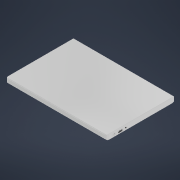
# Autodesk Inventor part: Razor Book 13
Saved by Autodesk Inventor 2021.3 (Build 253353000, 353)
## iProperties
Created: 2021-04-25
Part Number: Razor Book 13
Material: Generic
Document SubType Name: Modeling
Designer: trl121
Density: 1 g/cm^3
Appearance: Default
Author: trl121
Autodesk Inventor part; units mm, degrees
ref_plane "YZ Plane" through (0, 0, 0) normal (1, 0, 0) x (0, 1, 0)
ref_plane "XZ Plane" through (0, 0, 0) normal (0, 1, 0) x (-1, 0, 0)
ref_plane "XY Plane" through (0, 0, 0) normal (0, 0, 1) x (1, 0, 0)
sketch "Base" plane through (0, 0, 0) normal (0, 1, 0) x (-1, 0, 0)
  line L0 (-147.8, 99.5763) -> (147.8, 99.5763) construction
  line L1 (147.8, 99.5763) -> (147.8, -99.5763) construction
  line L2 (147.8, -99.5763) -> (-147.8, -99.5763) construction
  line L3 (-147.8, -99.5763) -> (-147.8, 99.5763) construction
  line L4 (-147.8, 99.5763) -> (147.8, 99.5763)
  line L5 (147.8, 99.5763) -> (147.8, -99.5763)
  line L6 (147.8, -99.5763) -> (-147.8, -99.5763)
  line L7 (-147.8, -99.5763) -> (-147.8, 99.5763)
  line L8 (-147.8, 99.5763) -> (147.8, -99.5763) construction
  line L9 (147.8, 99.5763) -> (-147.8, -99.5763) construction
  point P0 (0, 0)
  point P1 (0, 0)
  point P2 (0, 0)
  dimension "d2" = 295.6
  dimension "d6" = 199.1527
  constraints: 12 end point, 3 midpoint, 2 coincident, 2 horizontal, 2 parallel, 1 perpendicular, 2 other
  measures "d2" distance between parallel lines of L3 L1
  measures "d6" distance of L2.end L0.start
sketch "Side" plane through (0, 0, 0) normal (1, 0, 0) x (0, 1, 0)
  line L0 (0, -99.5763) -> (0, 99.5763) construction
  line L1 (7.8769, 99.5763) -> (7.8769, -99.5763) construction
  line L2 (7.8769, -99.5763) -> (-7.8769, -99.5763) construction
  line L3 (-7.8769, -99.5763) -> (-7.8769, 99.5763) construction
  line L4 (-7.8769, 99.5763) -> (7.8769, 99.5763) construction
  line L5 (7.8769, 99.5763) -> (-7.8769, 99.5763) construction
  line L6 (-7.8769, 99.5763) -> (-7.8769, -99.5763) construction
  line L7 (-7.8769, -99.5763) -> (7.8769, -99.5763) construction
  line L8 (7.8769, -99.5763) -> (7.8769, 99.5763) construction
  line L9 (6.5964, 99.5763) -> (6.5964, 98.1719)
  line L10 (6.5964, 98.1719) -> (7.8769, 98.1719)
  line L11 (-3.3255, 99.5763) -> (-3.3255, 98.1719)
  line L12 (-3.3255, 98.1719) -> (-4.3415, 98.1719)
  ellipse E0 centre (-4.3415, 88.4565) end of major axis (-4.3415, 98.1719) minor radius 2.4965 (-4.3415, 98.1719) -> (-6.838, 88.4565) ccw
  line L13 (-6.838, 88.4565) -> (-6.838, 75.8385)
  line L14 (6.5964, 99.5763) -> (-3.3255, 99.5763)
  ellipse E1 centre (-6.838, 74.0859) end of major axis (-6.838, 75.8385) minor radius 1.0389 (-6.838, 75.8385) -> (-7.8769, 74.0859) ccw
  line L15 (-6.838, 75.8385) -> (-6.308, 75.8385) construction
  line L16 (-7.8769, 74.0859) -> (-7.8769, 69.5647)
  line L17 (-7.8769, 71.8253) -> (-6.4493, 71.8253) construction
  ellipse E2 centre (-6.838, 69.5647) end of major axis (-6.838, 67.8121) minor radius 1.0389 (-7.8769, 69.5647) -> (-6.838, 67.8121) ccw
  line L18 (-6.838, 75.8385) -> (-6.838, 67.8121)
  line L19 (-6.838, 67.8121) -> (-6.838, -69.2956)
  line L20 (-6.838, -0.7418) -> (-5.3966, -0.7418) construction
  ellipse E3 centre (-6.838, -75.5694) end of major axis (-6.838, -77.322) minor radius 1.0389 (-7.8769, -75.5694) -> (-6.838, -77.322) ccw
  line L21 (-7.8769, -75.5694) -> (-7.8769, -71.0482)
  ellipse E4 centre (-6.838, -71.0482) end of major axis (-6.838, -69.2956) minor radius 1.0389 (-6.838, -69.2956) -> (-7.8769, -71.0482) ccw
  line L22 (-6.838, -77.322) -> (-6.838, -69.2956)
  line L23 (7.8769, 98.1719) -> (7.8769, -99.0683)
  line L24 (7.3689, -99.5763) -> (-4.2591, -99.5763)
  line L25 (-6.838, -77.322) -> (-6.838, -91.1477)
  ellipse E5 centre (-4.2591, -91.1477) end of major axis (-4.2591, -99.5763) minor radius 2.5789 (-6.838, -91.1477) -> (-4.2591, -99.5763) ccw
  arc A0 (7.3689, -99.5763) -> (7.8769, -99.0683) centre (7.3689, -99.0683) ccw
  point P0 (0, 0)
  point P1 (-5.6451, -98.2557)
  dimension "d42" = 1.016
  dimension "d82" = 1.7526
  dimension "d90" = 8.0264
  dimension "d119" = 0.508
  constraints: 42 end point, 13 horizontal, 11 point on line, 7 symmetric about line, 7 vertical, 6 perpendicular, 4 midpoint, 3 parallel, 2 collinear, 2 point on circle, 2 tangent, 1 centre point, 1 horizontal alignment, 28 other
  measures "d42" distance of L11.end L12.end
  measures "d82" distance from line of L15 point (-6.838, 74.086)
  measures "d90" distance from line of L18.end L15
  measures "d119" radius of A0
extrude "Main Body" add sketch "Side" along normal mid plane 295.6 contours L9 L10 L23 A0 L24 E5 L25 L22 L19 L18 L13 E0 L12 L11 L14
sketch "Bottom" plane through (-147.8, -6.838, -91.1477) normal (0, -1, 0) x (1, 0, 0)
  line L0 (0, 190.724) -> (295.6, 190.724) construction
  line L1 (295.6, 190.724) -> (295.6, 44.5306) construction
  line L2 (295.6, 44.5306) -> (0, 44.5306) construction
  line L3 (0, 44.5306) -> (0, 190.724) construction
  line L4 (295.6, 179.6042) -> (295.6, 0) projected
  line L5 (27.94, 140.178) -> (72.39, 140.178)
  line L6 (73.66, 138.908) -> (73.66, 135.606)
  line L7 (72.39, 134.336) -> (27.94, 134.336)
  line L8 (26.67, 135.606) -> (26.67, 138.908)
  arc A0 (27.94, 140.178) -> (26.67, 138.908) centre (27.94, 138.908) ccw
  arc A1 (26.67, 135.606) -> (27.94, 134.336) centre (27.94, 135.606) ccw
  arc A2 (73.66, 138.908) -> (72.39, 140.178) centre (72.39, 138.908) ccw
  arc A3 (72.39, 134.336) -> (73.66, 135.606) centre (72.39, 135.606) ccw
  line L9 (27.94, 130.78) -> (72.39, 130.78)
  arc A4 (27.94, 130.78) -> (26.67, 129.51) centre (27.94, 129.51) ccw
  line L10 (26.67, 126.208) -> (26.67, 129.51)
  arc A5 (26.67, 126.208) -> (27.94, 124.938) centre (27.94, 126.208) ccw
  line L11 (72.39, 124.938) -> (27.94, 124.938)
  arc A6 (72.39, 124.938) -> (73.66, 126.208) centre (72.39, 126.208) ccw
  line L12 (73.66, 129.51) -> (73.66, 126.208)
  arc A7 (73.66, 129.51) -> (72.39, 130.78) centre (72.39, 129.51) ccw
  line L13 (27.94, 121.382) -> (72.39, 121.382)
  arc A8 (27.94, 121.382) -> (26.67, 120.112) centre (27.94, 120.112) ccw
  line L14 (26.67, 116.81) -> (26.67, 120.112)
  arc A9 (26.67, 116.81) -> (27.94, 115.54) centre (27.94, 116.81) ccw
  line L15 (72.39, 115.54) -> (27.94, 115.54)
  arc A10 (72.39, 115.54) -> (73.66, 116.81) centre (72.39, 116.81) ccw
  line L16 (73.66, 120.112) -> (73.66, 116.81)
  arc A11 (73.66, 120.112) -> (72.39, 121.382) centre (72.39, 120.112) ccw
  line L17 (27.94, 111.984) -> (72.39, 111.984)
  arc A12 (27.94, 111.984) -> (26.67, 110.714) centre (27.94, 110.714) ccw
  line L18 (26.67, 107.412) -> (26.67, 110.714)
  arc A13 (26.67, 107.412) -> (27.94, 106.142) centre (27.94, 107.412) ccw
  line L19 (72.39, 106.142) -> (27.94, 106.142)
  arc A14 (72.39, 106.142) -> (73.66, 107.412) centre (72.39, 107.412) ccw
  line L20 (73.66, 110.714) -> (73.66, 107.412)
  arc A15 (73.66, 110.714) -> (72.39, 111.984) centre (72.39, 110.714) ccw
  line L21 (147.8, 190.724) -> (147.8, 44.5306) construction
  line L22 (267.66, 140.178) -> (223.21, 140.178)
  line L23 (221.94, 138.908) -> (221.94, 135.606)
  line L24 (223.21, 134.336) -> (267.66, 134.336)
  line L25 (268.93, 135.606) -> (268.93, 138.908)
  arc A16 (268.93, 138.908) -> (267.66, 140.178) centre (267.66, 138.908) ccw
  arc A17 (267.66, 134.336) -> (268.93, 135.606) centre (267.66, 135.606) ccw
  arc A18 (223.21, 140.178) -> (221.94, 138.908) centre (223.21, 138.908) ccw
  arc A19 (221.94, 135.606) -> (223.21, 134.336) centre (223.21, 135.606) ccw
  line L26 (267.66, 130.78) -> (223.21, 130.78)
  arc A20 (268.93, 129.51) -> (267.66, 130.78) centre (267.66, 129.51) ccw
  line L27 (268.93, 126.208) -> (268.93, 129.51)
  arc A21 (267.66, 124.938) -> (268.93, 126.208) centre (267.66, 126.208) ccw
  line L28 (223.21, 124.938) -> (267.66, 124.938)
  arc A22 (221.94, 126.208) -> (223.21, 124.938) centre (223.21, 126.208) ccw
  line L29 (221.94, 129.51) -> (221.94, 126.208)
  arc A23 (223.21, 130.78) -> (221.94, 129.51) centre (223.21, 129.51) ccw
  line L30 (267.66, 121.382) -> (223.21, 121.382)
  arc A24 (268.93, 120.112) -> (267.66, 121.382) centre (267.66, 120.112) ccw
  line L31 (268.93, 116.81) -> (268.93, 120.112)
  arc A25 (267.66, 115.54) -> (268.93, 116.81) centre (267.66, 116.81) ccw
  line L32 (223.21, 115.54) -> (267.66, 115.54)
  arc A26 (221.94, 116.81) -> (223.21, 115.54) centre (223.21, 116.81) ccw
  line L33 (221.94, 120.112) -> (221.94, 116.81)
  arc A27 (223.21, 121.382) -> (221.94, 120.112) centre (223.21, 120.112) ccw
  line L34 (267.66, 111.984) -> (223.21, 111.984)
  arc A28 (268.93, 110.714) -> (267.66, 111.984) centre (267.66, 110.714) ccw
  line L35 (268.93, 107.412) -> (268.93, 110.714)
  arc A29 (267.66, 106.142) -> (268.93, 107.412) centre (267.66, 107.412) ccw
  line L36 (223.21, 106.142) -> (267.66, 106.142)
  arc A30 (221.94, 107.412) -> (223.21, 106.142) centre (223.21, 107.412) ccw
  line L37 (221.94, 110.714) -> (221.94, 107.412)
  arc A31 (223.21, 111.984) -> (221.94, 110.714) centre (223.21, 110.714) ccw
  line L38 (0, 190.724) -> (295.6, 190.724) projected
  line L39 (5.08, 190.724) -> (0, 190.724)
  line L40 (0, 190.724) -> (0, 185.644)
  line L41 (0, 189.3196) -> (0, 179.6042) projected
  arc A32 (5.08, 190.724) -> (0, 185.644) centre (5.08, 185.644) ccw
  line L42 (295.6, 190.724) -> (295.6, 185.644)
  arc A33 (295.6, 185.644) -> (290.52, 190.724) centre (290.52, 185.644) ccw
  line L43 (290.52, 190.724) -> (295.6, 190.724)
  line L44 (27.5437, 176.5) -> (32.6237, 176.5)
  line L45 (33.1317, 175.992) -> (33.1317, 172.69)
  line L46 (32.6237, 172.182) -> (27.5437, 172.182)
  line L47 (27.0357, 172.69) -> (27.0357, 175.992)
  arc A34 (27.5437, 176.5) -> (27.0357, 175.992) centre (27.5437, 175.992) ccw
  arc A35 (27.0357, 172.69) -> (27.5437, 172.182) centre (27.5437, 172.69) ccw
  arc A36 (32.6237, 172.182) -> (33.1317, 172.69) centre (32.6237, 172.69) ccw
  arc A37 (33.1317, 175.992) -> (32.6237, 176.5) centre (32.6237, 175.992) ccw
  line L48 (37.7799, 176.5) -> (42.8599, 176.5)
  arc A38 (37.7799, 176.5) -> (37.2719, 175.992) centre (37.7799, 175.992) ccw
  line L49 (37.2719, 172.69) -> (37.2719, 175.992)
  arc A39 (37.2719, 172.69) -> (37.7799, 172.182) centre (37.7799, 172.69) ccw
  line L50 (42.8599, 172.182) -> (37.7799, 172.182)
  arc A40 (42.8599, 172.182) -> (43.3679, 172.69) centre (42.8599, 172.69) ccw
  line L51 (43.3679, 175.992) -> (43.3679, 172.69)
  arc A41 (43.3679, 175.992) -> (42.8599, 176.5) centre (42.8599, 175.992) ccw
  line L52 (48.0161, 176.5) -> (53.0961, 176.5)
  arc A42 (48.0161, 176.5) -> (47.5081, 175.992) centre (48.0161, 175.992) ccw
  line L53 (47.5081, 172.69) -> (47.5081, 175.992)
  arc A43 (47.5081, 172.69) -> (48.0161, 172.182) centre (48.0161, 172.69) ccw
  line L54 (53.0961, 172.182) -> (48.0161, 172.182)
  arc A44 (53.0961, 172.182) -> (53.6041, 172.69) centre (53.0961, 172.69) ccw
  line L55 (53.6041, 175.992) -> (53.6041, 172.69)
  arc A45 (53.6041, 175.992) -> (53.0961, 176.5) centre (53.0961, 175.992) ccw
  line L56 (58.2523, 176.5) -> (63.3323, 176.5)
  arc A46 (58.2523, 176.5) -> (57.7443, 175.992) centre (58.2523, 175.992) ccw
  line L57 (57.7443, 172.69) -> (57.7443, 175.992)
  arc A47 (57.7443, 172.69) -> (58.2523, 172.182) centre (58.2523, 172.69) ccw
  line L58 (63.3323, 172.182) -> (58.2523, 172.182)
  arc A48 (63.3323, 172.182) -> (63.8403, 172.69) centre (63.3323, 172.69) ccw
  line L59 (63.8403, 175.992) -> (63.8403, 172.69)
  arc A49 (63.8403, 175.992) -> (63.3323, 176.5) centre (63.3323, 175.992) ccw
  line L60 (68.4885, 176.5) -> (73.5685, 176.5)
  arc A50 (68.4885, 176.5) -> (67.9805, 175.992) centre (68.4885, 175.992) ccw
  line L61 (67.9805, 172.69) -> (67.9805, 175.992)
  arc A51 (67.9805, 172.69) -> (68.4885, 172.182) centre (68.4885, 172.69) ccw
  line L62 (73.5685, 172.182) -> (68.4885, 172.182)
  arc A52 (73.5685, 172.182) -> (74.0765, 172.69) centre (73.5685, 172.69) ccw
  line L63 (74.0765, 175.992) -> (74.0765, 172.69)
  arc A53 (74.0765, 175.992) -> (73.5685, 176.5) centre (73.5685, 175.992) ccw
  line L64 (78.7247, 176.5) -> (83.8047, 176.5)
  arc A54 (78.7247, 176.5) -> (78.2167, 175.992) centre (78.7247, 175.992) ccw
  line L65 (78.2167, 172.69) -> (78.2167, 175.992)
  arc A55 (78.2167, 172.69) -> (78.7247, 172.182) centre (78.7247, 172.69) ccw
  line L66 (83.8047, 172.182) -> (78.7247, 172.182)
  arc A56 (83.8047, 172.182) -> (84.3127, 172.69) centre (83.8047, 172.69) ccw
  line L67 (84.3127, 175.992) -> (84.3127, 172.69)
  arc A57 (84.3127, 175.992) -> (83.8047, 176.5) centre (83.8047, 175.992) ccw
  line L68 (88.9609, 176.5) -> (94.0409, 176.5) construction
  arc A58 (88.9609, 176.5) -> (88.4529, 175.992) centre (88.9609, 175.992) ccw construction
  line L69 (88.4529, 172.69) -> (88.4529, 175.992) construction
  arc A59 (88.4529, 172.69) -> (88.9609, 172.182) centre (88.9609, 172.69) ccw construction
  line L70 (94.0409, 172.182) -> (88.9609, 172.182) construction
  arc A60 (94.0409, 172.182) -> (94.5489, 172.69) centre (94.0409, 172.69) ccw construction
  line L71 (94.5489, 175.992) -> (94.5489, 172.69) construction
  arc A61 (94.5489, 175.992) -> (94.0409, 176.5) centre (94.0409, 175.992) ccw construction
  line L72 (99.1971, 176.5) -> (104.2771, 176.5)
  arc A62 (99.1971, 176.5) -> (98.6891, 175.992) centre (99.1971, 175.992) ccw
  line L73 (98.6891, 172.69) -> (98.6891, 175.992)
  arc A63 (98.6891, 172.69) -> (99.1971, 172.182) centre (99.1971, 172.69) ccw
  line L74 (104.2771, 172.182) -> (99.1971, 172.182)
  arc A64 (104.2771, 172.182) -> (104.7851, 172.69) centre (104.2771, 172.69) ccw
  line L75 (104.7851, 175.992) -> (104.7851, 172.69)
  arc A65 (104.7851, 175.992) -> (104.2771, 176.5) centre (104.2771, 175.992) ccw
  line L76 (109.4333, 176.5) -> (114.5133, 176.5)
  arc A66 (109.4333, 176.5) -> (108.9253, 175.992) centre (109.4333, 175.992) ccw
  line L77 (108.9253, 172.69) -> (108.9253, 175.992)
  arc A67 (108.9253, 172.69) -> (109.4333, 172.182) centre (109.4333, 172.69) ccw
  line L78 (114.5133, 172.182) -> (109.4333, 172.182)
  arc A68 (114.5133, 172.182) -> (115.0213, 172.69) centre (114.5133, 172.69) ccw
  line L79 (115.0213, 175.992) -> (115.0213, 172.69)
  arc A69 (115.0213, 175.992) -> (114.5133, 176.5) centre (114.5133, 175.992) ccw
  line L80 (119.6695, 176.5) -> (124.7495, 176.5)
  arc A70 (119.6695, 176.5) -> (119.1615, 175.992) centre (119.6695, 175.992) ccw
  line L81 (119.1615, 172.69) -> (119.1615, 175.992)
  arc A71 (119.1615, 172.69) -> (119.6695, 172.182) centre (119.6695, 172.69) ccw
  line L82 (124.7495, 172.182) -> (119.6695, 172.182)
  arc A72 (124.7495, 172.182) -> (125.2575, 172.69) centre (124.7495, 172.69) ccw
  line L83 (125.2575, 175.992) -> (125.2575, 172.69)
  arc A73 (125.2575, 175.992) -> (124.7495, 176.5) centre (124.7495, 175.992) ccw
  line L84 (129.9057, 176.5) -> (134.9857, 176.5)
  arc A74 (129.9057, 176.5) -> (129.3977, 175.992) centre (129.9057, 175.992) ccw
  line L85 (129.3977, 172.69) -> (129.3977, 175.992)
  arc A75 (129.3977, 172.69) -> (129.9057, 172.182) centre (129.9057, 172.69) ccw
  line L86 (134.9857, 172.182) -> (129.9057, 172.182)
  arc A76 (134.9857, 172.182) -> (135.4937, 172.69) centre (134.9857, 172.69) ccw
  line L87 (135.4937, 175.992) -> (135.4937, 172.69)
  arc A77 (135.4937, 175.992) -> (134.9857, 176.5) centre (134.9857, 175.992) ccw
  line L88 (140.1419, 176.5) -> (145.2219, 176.5)
  arc A78 (140.1419, 176.5) -> (139.6339, 175.992) centre (140.1419, 175.992) ccw
  line L89 (139.6339, 172.69) -> (139.6339, 175.992)
  arc A79 (139.6339, 172.69) -> (140.1419, 172.182) centre (140.1419, 172.69) ccw
  line L90 (145.2219, 172.182) -> (140.1419, 172.182)
  arc A80 (145.2219, 172.182) -> (145.7299, 172.69) centre (145.2219, 172.69) ccw
  line L91 (145.7299, 175.992) -> (145.7299, 172.69)
  arc A81 (145.7299, 175.992) -> (145.2219, 176.5) centre (145.2219, 175.992) ccw
  line L92 (150.3781, 176.5) -> (155.4581, 176.5)
  arc A82 (150.3781, 176.5) -> (149.8701, 175.992) centre (150.3781, 175.992) ccw
  line L93 (149.8701, 172.69) -> (149.8701, 175.992)
  arc A83 (149.8701, 172.69) -> (150.3781, 172.182) centre (150.3781, 172.69) ccw
  line L94 (155.4581, 172.182) -> (150.3781, 172.182)
  arc A84 (155.4581, 172.182) -> (155.9661, 172.69) centre (155.4581, 172.69) ccw
  line L95 (155.9661, 175.992) -> (155.9661, 172.69)
  arc A85 (155.9661, 175.992) -> (155.4581, 176.5) centre (155.4581, 175.992) ccw
  line L96 (160.6143, 176.5) -> (165.6943, 176.5)
  arc A86 (160.6143, 176.5) -> (160.1063, 175.992) centre (160.6143, 175.992) ccw
  line L97 (160.1063, 172.69) -> (160.1063, 175.992)
  arc A87 (160.1063, 172.69) -> (160.6143, 172.182) centre (160.6143, 172.69) ccw
  line L98 (165.6943, 172.182) -> (160.6143, 172.182)
  arc A88 (165.6943, 172.182) -> (166.2023, 172.69) centre (165.6943, 172.69) ccw
  line L99 (166.2023, 175.992) -> (166.2023, 172.69)
  arc A89 (166.2023, 175.992) -> (165.6943, 176.5) centre (165.6943, 175.992) ccw
  line L100 (170.8505, 176.5) -> (175.9305, 176.5)
  arc A90 (170.8505, 176.5) -> (170.3425, 175.992) centre (170.8505, 175.992) ccw
  line L101 (170.3425, 172.69) -> (170.3425, 175.992)
  arc A91 (170.3425, 172.69) -> (170.8505, 172.182) centre (170.8505, 172.69) ccw
  line L102 (175.9305, 172.182) -> (170.8505, 172.182)
  arc A92 (175.9305, 172.182) -> (176.4385, 172.69) centre (175.9305, 172.69) ccw
  line L103 (176.4385, 175.992) -> (176.4385, 172.69)
  arc A93 (176.4385, 175.992) -> (175.9305, 176.5) centre (175.9305, 175.992) ccw
  line L104 (181.0867, 176.5) -> (186.1667, 176.5)
  arc A94 (181.0867, 176.5) -> (180.5787, 175.992) centre (181.0867, 175.992) ccw
  line L105 (180.5787, 172.69) -> (180.5787, 175.992)
  arc A95 (180.5787, 172.69) -> (181.0867, 172.182) centre (181.0867, 172.69) ccw
  line L106 (186.1667, 172.182) -> (181.0867, 172.182)
  arc A96 (186.1667, 172.182) -> (186.6747, 172.69) centre (186.1667, 172.69) ccw
  line L107 (186.6747, 175.992) -> (186.6747, 172.69)
  arc A97 (186.6747, 175.992) -> (186.1667, 176.5) centre (186.1667, 175.992) ccw
  line L108 (191.3229, 176.5) -> (196.4029, 176.5)
  arc A98 (191.3229, 176.5) -> (190.8149, 175.992) centre (191.3229, 175.992) ccw
  line L109 (190.8149, 172.69) -> (190.8149, 175.992)
  arc A99 (190.8149, 172.69) -> (191.3229, 172.182) centre (191.3229, 172.69) ccw
  line L110 (196.4029, 172.182) -> (191.3229, 172.182)
  arc A100 (196.4029, 172.182) -> (196.9109, 172.69) centre (196.4029, 172.69) ccw
  line L111 (196.9109, 175.992) -> (196.9109, 172.69)
  arc A101 (196.9109, 175.992) -> (196.4029, 176.5) centre (196.4029, 175.992) ccw
  line L112 (201.5591, 176.5) -> (206.6391, 176.5) construction
  arc A102 (201.5591, 176.5) -> (201.0511, 175.992) centre (201.5591, 175.992) ccw construction
  line L113 (201.0511, 172.69) -> (201.0511, 175.992) construction
  arc A103 (201.0511, 172.69) -> (201.5591, 172.182) centre (201.5591, 172.69) ccw construction
  line L114 (206.6391, 172.182) -> (201.5591, 172.182) construction
  arc A104 (206.6391, 172.182) -> (207.1471, 172.69) centre (206.6391, 172.69) ccw construction
  line L115 (207.1471, 175.992) -> (207.1471, 172.69) construction
  arc A105 (207.1471, 175.992) -> (206.6391, 176.5) centre (206.6391, 175.992) ccw construction
  line L116 (211.7953, 176.5) -> (216.8753, 176.5)
  arc A106 (211.7953, 176.5) -> (211.2873, 175.992) centre (211.7953, 175.992) ccw
  line L117 (211.2873, 172.69) -> (211.2873, 175.992)
  arc A107 (211.2873, 172.69) -> (211.7953, 172.182) centre (211.7953, 172.69) ccw
  line L118 (216.8753, 172.182) -> (211.7953, 172.182)
  arc A108 (216.8753, 172.182) -> (217.3833, 172.69) centre (216.8753, 172.69) ccw
  line L119 (217.3833, 175.992) -> (217.3833, 172.69)
  arc A109 (217.3833, 175.992) -> (216.8753, 176.5) centre (216.8753, 175.992) ccw
  line L120 (222.0315, 176.5) -> (227.1115, 176.5)
  arc A110 (222.0315, 176.5) -> (221.5235, 175.992) centre (222.0315, 175.992) ccw
  line L121 (221.5235, 172.69) -> (221.5235, 175.992)
  arc A111 (221.5235, 172.69) -> (222.0315, 172.182) centre (222.0315, 172.69) ccw
  line L122 (227.1115, 172.182) -> (222.0315, 172.182)
  arc A112 (227.1115, 172.182) -> (227.6195, 172.69) centre (227.1115, 172.69) ccw
  line L123 (227.6195, 175.992) -> (227.6195, 172.69)
  arc A113 (227.6195, 175.992) -> (227.1115, 176.5) centre (227.1115, 175.992) ccw
  line L124 (232.2677, 176.5) -> (237.3477, 176.5)
  arc A114 (232.2677, 176.5) -> (231.7597, 175.992) centre (232.2677, 175.992) ccw
  line L125 (231.7597, 172.69) -> (231.7597, 175.992)
  arc A115 (231.7597, 172.69) -> (232.2677, 172.182) centre (232.2677, 172.69) ccw
  line L126 (237.3477, 172.182) -> (232.2677, 172.182)
  arc A116 (237.3477, 172.182) -> (237.8557, 172.69) centre (237.3477, 172.69) ccw
  line L127 (237.8557, 175.992) -> (237.8557, 172.69)
  arc A117 (237.8557, 175.992) -> (237.3477, 176.5) centre (237.3477, 175.992) ccw
  line L128 (242.5039, 176.5) -> (247.5839, 176.5)
  arc A118 (242.5039, 176.5) -> (241.9959, 175.992) centre (242.5039, 175.992) ccw
  line L129 (241.9959, 172.69) -> (241.9959, 175.992)
  arc A119 (241.9959, 172.69) -> (242.5039, 172.182) centre (242.5039, 172.69) ccw
  line L130 (247.5839, 172.182) -> (242.5039, 172.182)
  arc A120 (247.5839, 172.182) -> (248.0919, 172.69) centre (247.5839, 172.69) ccw
  line L131 (248.0919, 175.992) -> (248.0919, 172.69)
  arc A121 (248.0919, 175.992) -> (247.5839, 176.5) centre (247.5839, 175.992) ccw
  line L132 (252.7401, 176.5) -> (257.8201, 176.5)
  arc A122 (252.7401, 176.5) -> (252.2321, 175.992) centre (252.7401, 175.992) ccw
  line L133 (252.2321, 172.69) -> (252.2321, 175.992)
  arc A123 (252.2321, 172.69) -> (252.7401, 172.182) centre (252.7401, 172.69) ccw
  line L134 (257.8201, 172.182) -> (252.7401, 172.182)
  arc A124 (257.8201, 172.182) -> (258.3281, 172.69) centre (257.8201, 172.69) ccw
  line L135 (258.3281, 175.992) -> (258.3281, 172.69)
  arc A125 (258.3281, 175.992) -> (257.8201, 176.5) centre (257.8201, 175.992) ccw
  line L136 (262.9763, 176.5) -> (268.0563, 176.5)
  arc A126 (262.9763, 176.5) -> (262.4683, 175.992) centre (262.9763, 175.992) ccw
  line L137 (262.4683, 172.69) -> (262.4683, 175.992)
  arc A127 (262.4683, 172.69) -> (262.9763, 172.182) centre (262.9763, 172.69) ccw
  line L138 (268.0563, 172.182) -> (262.9763, 172.182)
  arc A128 (268.0563, 172.182) -> (268.5643, 172.69) centre (268.0563, 172.69) ccw
  line L139 (268.5643, 175.992) -> (268.5643, 172.69)
  arc A129 (268.5643, 175.992) -> (268.0563, 176.5) centre (268.0563, 175.992) ccw
  point P0 (147.8, 91.1477)
  point P1 (26.67, 140.178)
  point P2 (73.66, 140.178)
  point P3 (26.67, 134.336)
  point P4 (26.67, 130.78)
  point P5 (73.66, 130.78)
  point P6 (26.67, 124.938)
  point P7 (26.67, 121.382)
  point P8 (73.66, 121.382)
  point P9 (26.67, 115.54)
  point P10 (26.67, 111.984)
  point P11 (73.66, 111.984)
  point P12 (26.67, 106.142)
  point P13 (27.0357, 176.5)
  point P14 (33.1317, 172.182)
  point P15 (27.0357, 172.182)
  point P16 (37.2719, 176.5)
  point P17 (37.2719, 172.182)
  point P18 (43.3679, 172.182)
  point P19 (47.5081, 176.5)
  point P20 (47.5081, 172.182)
  point P21 (53.6041, 172.182)
  point P22 (57.7443, 176.5)
  point P23 (57.7443, 172.182)
  point P24 (63.8403, 172.182)
  point P25 (67.9805, 176.5)
  point P26 (67.9805, 172.182)
  point P27 (74.0765, 172.182)
  point P28 (78.2167, 176.5)
  point P29 (78.2167, 172.182)
  point P30 (84.3127, 172.182)
  point P31 (88.4529, 176.5)
  point P32 (88.4529, 172.182)
  point P33 (94.5489, 172.182)
  point P34 (98.6891, 176.5)
  point P35 (98.6891, 172.182)
  point P36 (104.7851, 172.182)
  point P37 (108.9253, 176.5)
  point P38 (108.9253, 172.182)
  point P39 (115.0213, 172.182)
  point P40 (119.1615, 176.5)
  point P41 (119.1615, 172.182)
  point P42 (125.2575, 172.182)
  point P43 (129.3977, 176.5)
  point P44 (129.3977, 172.182)
  point P45 (135.4937, 172.182)
  point P46 (139.6339, 176.5)
  point P47 (139.6339, 172.182)
  point P48 (145.7299, 172.182)
  point P49 (149.8701, 176.5)
  point P50 (149.8701, 172.182)
  point P51 (155.9661, 172.182)
  point P52 (160.1063, 176.5)
  point P53 (160.1063, 172.182)
  point P54 (166.2023, 172.182)
  point P55 (170.3425, 176.5)
  point P56 (170.3425, 172.182)
  point P57 (176.4385, 172.182)
  point P58 (180.5787, 176.5)
  point P59 (180.5787, 172.182)
  point P60 (186.6747, 172.182)
  point P61 (190.8149, 176.5)
  point P62 (190.8149, 172.182)
  point P63 (196.9109, 172.182)
  point P64 (201.0511, 176.5)
  point P65 (201.0511, 172.182)
  point P66 (207.1471, 172.182)
  point P67 (211.2873, 176.5)
  point P68 (211.2873, 172.182)
  point P69 (217.3833, 172.182)
  point P70 (221.5235, 176.5)
  point P71 (221.5235, 172.182)
  point P72 (227.6195, 172.182)
  point P73 (231.7597, 176.5)
  point P74 (231.7597, 172.182)
  point P75 (237.8557, 172.182)
  point P76 (241.9959, 176.5)
  point P77 (241.9959, 172.182)
  point P78 (248.0919, 172.182)
  point P79 (252.2321, 176.5)
  point P80 (252.2321, 172.182)
  point P81 (258.3281, 172.182)
  point P82 (262.4683, 176.5)
  point P83 (262.4683, 172.182)
  point P84 (268.5643, 172.182)
  dimension "d149" = 46.99
  dimension "d150" = 5.842
  dimension "d151" = 26.67
  dimension "d153" = 50.546
  dimension "d154" = 1.27
  dimension "d165" = 9.398
  dimension "d182" = 5.08
  dimension "d189" = 4.318
  dimension "d191" = 6.096
  dimension "d192" = 0.508
  dimension "d202" = 14.224
  dimension "d207" = 10.2362
  constraints: 267 end point, 260 point on circle, 170 point on line, 130 centre point, 52 symmetric about line, 19 tangent, 6 equal radius, 4 collinear, 4 parallel, 3 horizontal, 2 midpoint, 2 perpendicular, 1 coincident, 1 vertical, 618 other
  measures "d149" distance of point (26.67, 140.178) point (73.66, 140.178)
  measures "d150" distance of point (26.67, 134.336) point (26.67, 140.178)
  measures "d151" distance between parallel lines of L3 L8
  measures "d153" distance between parallel lines of L0 L5
  measures "d154" radius of A0
  measures "d165" distance of L5.start L9.start
  measures "d182" radius of A32
  measures "d189" distance of point (27.036, 172.182) point (27.036, 176.5)
  measures "d191" distance of point (33.132, 172.182) point (27.036, 172.182)
  measures "d192" radius of A34
  measures "d202" distance between parallel lines of L44 L38
  measures "d207" distance of L44.start L48.start
extrude "MainLeg" add sketch "Side" along normal mid plane 237.4948 contours L18 E2 L16 E1 | E3 L21 E4 L22
sketch "Leg Ends" plane through (-118.7474, 0, 0) normal (-1, 0, 0) x (0, 0, 1)
  ellipse E0 centre (74.0859, -6.838) end of major axis (75.8385, -6.838) minor radius 1.0389 (74.0859, -7.8769) -> (75.8385, -6.838) ccw projected
  ellipse E1 centre (69.5647, -6.838) end of major axis (67.8121, -6.838) minor radius 1.0389 (67.8121, -6.838) -> (69.5647, -7.8769) ccw projected
  line L0 (-91.1477, -6.838) -> (88.4565, -6.838) projected
  line L1 (69.5647, -7.8769) -> (69.5647, -6.838)
  line L2 (88.4565, -6.838) -> (-91.1477, -6.838) projected
  line L3 (74.0859, -7.8769) -> (74.0859, -6.838)
  ellipse E2 centre (-71.0482, -6.838) end of major axis (-69.2956, -6.838) minor radius 1.0389 (-71.0482, -7.8769) -> (-69.2956, -6.838) ccw projected
  ellipse E3 centre (-75.5694, -6.838) end of major axis (-77.322, -6.838) minor radius 1.0389 (-77.322, -6.838) -> (-75.5694, -7.8769) ccw projected
  line L4 (-71.0482, -7.8769) -> (-71.0482, -6.838)
  line L5 (-75.5694, -7.8769) -> (-75.5694, -6.838)
  point P0 (0, 0)
  constraints: 8 end point, 3 vertical, 1 perpendicular, 4 other
revolve "Leg End Rev1" add sketch "Leg Ends" angle 90 about axis through (-118.7474, -7.8769, 74.0859) along (0, -1, 0) contours L3 L0 E0
revolve "Leg End Rev2" add sketch "Leg Ends" angle 90 about axis through (-118.7474, -7.8769, 69.5647) along (0, 1, 0) contours L1 E1 L0
revolve "Leg End Rev3" add sketch "Leg Ends" angle 90 about axis through (-118.7474, -7.8769, -75.5694) along (0, 1, 0) contours L5 E3 L0
revolve "Leg End Rev4" add sketch "Leg Ends" angle 90 about axis through (-118.7474, -7.8769, -71.0482) along (0, -1, 0) contours E2 L4 L0
sketch "Sketch5" plane through (-118.7474, -7.8769, 74.0859) normal (0, 0, -1) x (-1, 0, 0)
  ellipse E0 centre (0, 1.0389) end of major axis (1.7526, 1.0389) minor radius 1.0389 (0, 0) -> (1.7526, 1.0389) ccw projected
  line L0 (0, 1.0389) -> (1.7526, 1.0389) projected
  line L1 (0, 0) -> (0, 1.0389) projected
  point P0 (-118.7474, 7.8769)
  constraints: 1 other
extrude "Leg End 1" add sketch "Sketch5" along normal up to surface (4.5212 mm away)
sketch "Sketch6" plane through (-118.7474, -7.8769, -75.5694) normal (0, 0, 1) x (1, 0, 0)
  line L0 (-1.7526, 1.0389) -> (0, 1.0389) projected
  ellipse E0 centre (0, 1.0389) end of major axis (-1.7526, 1.0389) minor radius 1.0389 (-1.7526, 1.0389) -> (0, 0) ccw projected
  line L1 (0, 1.0389) -> (0, 0) projected
  point P0 (118.7474, 7.8769)
  constraints: 1 other
extrude "Leg End 2" add sketch "Sketch6" along normal up to surface (4.5212 mm away)
mirror "Leg Ends Mir" about plane through (0, 0, 0) normal (1, 0, 0) of "Leg End Rev1", "Leg End Rev2", "Leg End Rev3", "Leg End Rev4", "Leg End 1", "Leg End 2"
extrude "Intake Vents" cut sketch "Bottom" against normal blind 0.508 contours L5 A2 L6 A3 L7 A1 L8 A0 | L9 A7 L12 A6 L11 A5 L10 A4 | L13 A11 L16 A10 L15 A9 L14 A8 | L17 A15 L20 A14 L19 A13 L18 A12 | A16 L25 A17 L24 A19 L23 A18 L22 | A20 L27 A21 L28 A22 L29 A23 L26 | A24 L31 A25 L32 A26 L33 A27 L30 | A28 L35 A29 L36 A30 L37 A31 L34
extrude "Corner Bevels" cut sketch "Bottom" against normal through all contours L38 L42 A33 | L38 A32 L40
extrude "Exhaust Vents" cut sketch "Bottom" against normal blind 1.27 contours L44 A37 L45 A36 L46 A35 L47 A34 | L48 A41 L51 A40 L50 A39 L49 A38 | L52 A45 L55 A44 L54 A43 L53 A42 | L56 A49 L59 A48 L58 A47 L57 A46 | L60 A53 L63 A52 L62 A51 L61 A50 | L64 A57 L67 A56 L66 A55 L65 A54 | L72 A65 L75 A64 L74 A63 L73 A62 | L76 A69 L79 A68 L78 A67 L77 A66 | L80 A73 L83 A72 L82 A71 L81 A70 | L84 A77 L87 A76 L86 A75 L85 A74 | L88 A81 L91 A80 L90 A79 L89 A78 | L92 A85 L95 A84 L94 A83 L93 A82 | L96 A89 L99 A88 L98 A87 L97 A86 | L100 A93 L103 A92 L102 A91 L101 A90 | L104 A97 L107 A96 L106 A95 L105 A94 | L108 A101 L111 A100 L110 A99 L109 A98 | L116 A109 L119 A108 L118 A107 L117 A106 | L120 A113 L123 A112 L122 A111 L121 A110 | L124 A117 L127 A116 L126 A115 L125 A114 | L128 A121 L131 A120 L130 A119 L129 A118 | L132 A125 L135 A124 L134 A123 L133 A122 | L136 A129 L139 A128 L138 A127 L137 A126
sketch "Sketch7" plane through (147.8, 0, 0) normal (1, 0, 0) x (0, 0, -1)
  line L0 (-99.5763, 7.8769) -> (99.5763, 7.8769) construction
  line L1 (99.5763, 7.8769) -> (99.5763, -7.8769) construction
  line L2 (99.5763, -7.8769) -> (-99.5763, -7.8769) construction
  line L3 (-99.5763, -7.8769) -> (-99.5763, 7.8769) construction
  line L4 (99.0683, 7.8769) -> (-94.4963, 7.8769) construction
  line L5 (99.5763, -4.2591) -> (99.5763, 7.3689) construction
  line L6 (-99.5763, 6.5964) -> (-99.5763, -3.3255) construction
  line L7 (-79.4343, -1.5269) -> (-73.7443, -1.5269) construction
  line L8 (-79.4343, -2.8519) -> (-73.7443, -2.8519)
  line L9 (-73.7443, -0.2019) -> (-79.4343, -0.2019)
  arc A0 (-79.4343, -0.2019) -> (-79.4343, -2.8519) centre (-79.4343, -1.5269) ccw
  arc A1 (-73.7443, -2.8519) -> (-73.7443, -0.2019) centre (-73.7443, -1.5269) ccw
  line L10 (-79.9343, -1.8769) -> (-73.2443, -1.8769)
  line L11 (-73.2443, -1.8769) -> (-73.2443, -1.1769)
  line L12 (-73.2443, -1.1769) -> (-79.9343, -1.1769)
  line L13 (-79.9343, -1.1769) -> (-79.9343, -1.8769)
  line L14 (-79.9343, -1.8769) -> (-73.2443, -1.1769) construction
  line L15 (-73.2443, -1.8769) -> (-79.9343, -1.1769) construction
  line L16 (-64.7783, -4.0669) -> (-52.2783, -4.0669)
  line L17 (-52.2783, -4.0669) -> (-52.2783, 1.0531)
  line L18 (-52.2783, 1.0531) -> (-64.7783, 1.0531)
  line L19 (-64.7783, 1.0531) -> (-64.7783, -4.0669)
  line L20 (-64.7783, -4.0669) -> (-52.2783, 1.0531) construction
  line L21 (-52.2783, -4.0669) -> (-64.7783, 1.0531) construction
  line L22 (-53.3213, -1.7809) -> (-63.7353, -1.7809)
  line L23 (-63.7353, -1.7809) -> (-63.7353, -0.1807)
  line L24 (-63.7353, -0.1807) -> (-53.3213, -0.1807)
  line L25 (-53.3213, -0.1807) -> (-53.3213, -1.7809)
  line L26 (-53.3213, -1.7809) -> (-63.7353, -0.1807) construction
  line L27 (-63.7353, -1.7809) -> (-53.3213, -0.1807) construction
  circle A2 centre (-42.2993, -1.0189) radius 1.85
  point P0 (0, 0)
  point P1 (-76.5893, -1.5269)
  point P2 (-58.5283, -1.5069)
  point P3 (-58.5283, -0.9808)
  point P4 (-58.5283, -1.5069)
  point P5 (-58.5283, -0.9808)
  dimension "d235" = 8.34
  dimension "d236" = 2.65
  dimension "d237" = 6.35
  dimension "d239" = 22.987
  dimension "d240" = 6.69
  dimension "d241" = 0.7
  dimension "d242" = 5.12
  dimension "d243" = 12.5
  dimension "d246" = 3.81
  dimension "d248" = 34.798
  dimension "d252" = 10.414
  dimension "d254" = 1.6002
  dimension "d257" = 3.7
  dimension "d259" = 57.277
  dimension "d261" = 6.858
  dimension "d265" = 2.286
  constraints: 44 end point, 9 midpoint, 7 parallel, 4 horizontal, 4 point on circle, 4 tangent, 3 centre point, 3 collinear, 3 perpendicular, 1 vertical alignment, 2 other
  measures "d236" distance between parallel lines of L8 L9
  measures "d237" distance between parallel lines of L2 L7
  measures "d239" distance from line of L3 point (-76.589, -1.527)
  measures "d240" distance of L11.end L12.end
  measures "d241" distance of L10.end L11.end
  measures "d242" distance of L16.end L17.end
  measures "d243" distance of L17.end L18.end
  measures "d246" distance between parallel lines of L16 L2
  measures "d248" distance between parallel lines of L3 L19
  measures "d252" distance of L23.end L24.end
  measures "d254" distance of L24.end L22.start
  measures "d257" diameter of A2
  measures "d259" distance from line of L3 A2.centre
  measures "d261" distance from line of L2 A2.centre
  measures "d265" distance between parallel lines of L16 L22
extrude "Left Side Ports" cut sketch "Sketch7" against normal blind 5.08
sketch "Sketch8" plane through (-147.8, 0, 0) normal (-1, 0, 0) x (0, 0, 1)
  line L0 (-99.5763, 7.8769) -> (99.5456, 8.2566) construction
  line L1 (99.5456, 8.2566) -> (99.5763, -7.8769) construction
  line L2 (99.5763, -7.8769) -> (-99.5456, -8.2566) construction
  line L3 (-99.5456, -8.2566) -> (-99.5763, 7.8769) construction
  line L4 (94.4963, 7.8769) -> (-99.0683, 7.8769) construction
  line L5 (-99.5763, 7.3689) -> (-99.5763, -4.2591) construction
  line L6 (-75.5694, -7.8769) -> (-71.0482, -7.8769) construction
  line L7 (99.5763, 6.5964) -> (99.5763, -3.3255) construction
  line L8 (-99.0683, 7.8769) -> (94.4963, 7.8769) construction
  line L9 (-99.0683, 7.8769) -> (-99.5763, 7.8769) construction
  arc A0 (-99.0683, 7.8769) -> (-99.5763, 7.3689) centre (-99.0683, 7.3689) ccw construction
  line L10 (-99.5763, 7.8769) -> (-99.5763, 7.3689) construction
  line L11 (-71.0482, -7.8769) -> (-75.5694, -7.8769) construction
  line L12 (-71.0482, -7.8769) -> (99.5763, -7.8769) construction
  line L13 (99.5763, 6.5964) -> (99.5763, -3.3255) construction
  line L14 (99.5763, -7.8769) -> (99.5763, -3.3255) construction
  line L15 (33.0039, -1.5275) -> (44.1493, -1.5275) construction
  line L16 (33.0039, -2.0746) -> (44.1493, -2.0746)
  line L17 (44.1493, -0.9804) -> (33.0039, -0.9804)
  arc A1 (33.0039, -0.9804) -> (33.0039, -2.0746) centre (33.0039, -1.5275) ccw
  arc A2 (44.1493, -2.0746) -> (44.1493, -0.9804) centre (44.1493, -1.5275) ccw
  line L18 (73.6584, -1.6001) -> (79.7714, -1.6001) construction
  line L19 (73.6584, -2.9159) -> (79.7714, -2.9159)
  line L20 (79.7714, -0.2843) -> (73.6584, -0.2843)
  arc A3 (73.6584, -0.2843) -> (73.6584, -2.9159) centre (73.6584, -1.6001) ccw
  arc A4 (79.7714, -2.9159) -> (79.7714, -0.2843) centre (79.7714, -1.6001) ccw
  line L21 (58.6208, 0.669) -> (51.7168, 0.669)
  line L22 (51.7168, 0.669) -> (51.7168, -2.2496)
  line L23 (51.7168, -2.2496) -> (53.8963, -3.9959)
  line L24 (53.8963, -3.9959) -> (58.6208, -3.9959)
  line L25 (58.6208, -3.9959) -> (58.6208, 0.669) construction
  line L26 (58.6208, 0.669) -> (65.5248, 0.669)
  line L27 (65.5248, 0.669) -> (65.5248, -2.2496)
  line L28 (65.5248, -2.2496) -> (63.3453, -3.9959)
  line L29 (63.3453, -3.9959) -> (58.6208, -3.9959)
  line L30 (53.2477, -1.3354) -> (63.9939, -1.3354)
  line L31 (63.9939, -1.3354) -> (63.9939, -2.2496)
  line L32 (63.9939, -2.2496) -> (53.2477, -2.2496)
  line L33 (53.2477, -2.2496) -> (53.2477, -1.3354)
  line L34 (73.9449, -1.6001) -> (79.4849, -1.6001) construction
  line L35 (73.9449, -1.8737) -> (79.4849, -1.8737)
  line L36 (79.4849, -1.3265) -> (73.9449, -1.3265)
  arc A5 (73.9449, -1.3265) -> (73.9449, -1.8737) centre (73.9449, -1.6001) ccw
  arc A6 (79.4849, -1.8737) -> (79.4849, -1.3265) centre (79.4849, -1.6001) ccw
  point P0 (0, 0)
  point P1 (38.5766, -1.5275)
  point P2 (76.7149, -1.6001)
  point P3 (58.6208, -1.3354)
  point P4 (76.7149, -1.6001)
  constraints: 58 end point, 14 tangent, 12 point on circle, 9 horizontal, 6 centre point, 5 parallel, 5 perpendicular, 4 midpoint, 3 symmetric about line, 2 coincident, 1 point on line, 4 other
extrude "Right Side Ports" cut sketch "Sketch8" against normal blind 5.08
body "Solid1"
